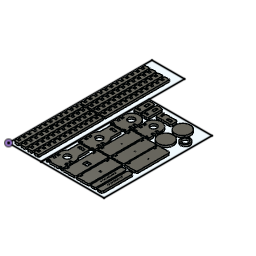
FinalFrameCAD (Autodesk Fusion 360 design; units mm, degrees)
Autodesk Fusion 360 part; units mm, degrees
note: some values were not read from the file. Chosen so that the rebuilt part matches the saved one: which bodies a step acts on.
sketch "Sketch1" plane through (0, 0, 0) normal (0, 0, 1) x (1, 0, 0)
  arc A0 (76.2, 342.8418) -> (-76.2, 342.8418) centre (0, 342.9) ccw
  line L0 (-45.085, 215.9582) -> (-45.085, 228.6582)
  line L1 (-45.085, 228.6582) -> (-63.5, 228.6582)
  line L2 (-63.5, 228.6582) -> (-63.5, 215.9582)
  line L3 (63.5, 215.9582) -> (63.5, 228.6582)
  line L4 (63.5, 228.6582) -> (45.085, 228.6582)
  line L5 (45.085, 228.6582) -> (45.085, 215.9582)
  line L6 (76.2, 215.9582) -> (63.5, 215.9582)
  line L7 (45.085, 215.9582) -> (-45.085, 215.9582)
  circle A1 centre (0, 342.9) radius 31.5595
  line L8 (76.2, 285.75) -> (50.8, 285.75)
  line L9 (50.8, 285.75) -> (50.8, 267.335)
  line L10 (50.8, 267.335) -> (76.2, 267.335)
  line L11 (76.2, 342.8418) -> (76.2, 323.85)
  line L12 (-76.2, 241.2418) -> (-76.2, 215.9582)
  line L13 (-76.2, 215.9582) -> (-63.5, 215.9582)
  line L14 (76.2, 305.435) -> (76.2, 285.75)
  line L15 (76.2, 267.335) -> (76.2, 215.9582)
  line L16 (76.2, 323.85) -> (50.8, 323.85)
  line L17 (50.8, 323.85) -> (50.8, 305.435)
  line L18 (50.8, 305.435) -> (76.2, 305.435)
  line L19 (-76.2, 323.85) -> (-50.8, 323.85)
  line L20 (-50.8, 323.85) -> (-50.8, 305.435)
  line L21 (-50.8, 305.435) -> (-76.2, 305.435)
  line L22 (-76.2, 285.75) -> (-50.8, 285.75)
  line L23 (-50.8, 285.75) -> (-50.8, 267.335)
  line L24 (-50.8, 267.335) -> (-76.2, 267.335)
  line L25 (-76.2, 323.85) -> (-76.2, 342.8418)
  line L26 (-76.2, 241.2418) -> (-76.2, 267.335)
  line L27 (-76.2, 285.75) -> (-76.2, 305.435)
  line L28 (279.4, 819.15) -> (254, 819.15)
  line L29 (266.7, 762.0582) -> (248.285, 762.0582)
  circle A2 centre (203.2, 876.3) radius 31.5595
  line L30 (254, 800.735) -> (279.4, 800.735)
  line L31 (279.4, 876.2418) -> (279.4, 857.25)
  line L32 (127, 749.3582) -> (139.7, 749.3582)
  line L33 (248.285, 762.0582) -> (248.285, 749.3582)
  line L34 (279.4, 857.25) -> (254, 857.25)
  line L35 (248.285, 749.3582) -> (158.115, 749.3582)
  line L36 (279.4, 838.835) -> (279.4, 819.15)
  line L37 (279.4, 800.735) -> (279.4, 749.3582)
  line L38 (254, 857.25) -> (254, 838.835)
  line L39 (254, 819.15) -> (254, 800.735)
  line L40 (152.4, 819.15) -> (152.4, 800.735)
  line L41 (127, 774.6418) -> (127, 749.3582)
  line L42 (152.4, 857.25) -> (152.4, 838.835)
  line L43 (139.7, 762.0582) -> (139.7, 749.3582)
  line L44 (158.115, 749.3582) -> (158.115, 762.0582)
  line L45 (127, 857.25) -> (127, 876.2418)
  line L46 (127, 819.15) -> (152.4, 819.15)
  line L47 (127, 819.15) -> (127, 838.835)
  line L48 (279.4, 749.3582) -> (266.7, 749.3582)
  line L49 (158.115, 762.0582) -> (139.7, 762.0582)
  line L50 (266.7, 749.3582) -> (266.7, 762.0582)
  line L51 (127, 857.25) -> (152.4, 857.25)
  line L52 (152.4, 838.835) -> (127, 838.835)
  line L53 (152.4, 800.735) -> (127, 800.735)
  line L54 (127, 774.6418) -> (127, 800.735)
  line L55 (254, 838.835) -> (279.4, 838.835)
  line L56 (203.2, 1003.1095) -> (228.6, 1003.1095)
  line L57 (228.6, 1003.1095) -> (228.6, 1021.5245)
  line L58 (228.6, 1021.5245) -> (203.2, 1021.5245)
  line L59 (177.8, 1021.5245) -> (203.2, 1021.5245)
  line L60 (203.2, 1003.1095) -> (177.8, 1003.1095)
  line L61 (177.8, 1003.1095) -> (177.8, 1021.5245)
  line L62 (152.4, 1021.5245) -> (152.4, 933.0961)
  line L63 (254, 1021.5245) -> (254, 933.0961)
  line L64 (152.4, 1021.5245) -> (152.4, 1046.9245)
  line L65 (152.4, 1046.9245) -> (254, 1046.9245)
  line L66 (254, 1046.9245) -> (254, 1021.5245)
  arc A3 (279.4, 876.2418) -> (254, 933.0961) centre (203.2, 876.3) ccw
  arc A4 (152.4, 933.0961) -> (127, 876.2418) centre (203.2, 876.3) ccw
  line L67 (590.55, 1066.8) -> (730.25, 1066.8)
  line L68 (812.8, 1066.8) -> (812.8, 1016)
  line L69 (812.8, 1016) -> (508, 1016)
  line L70 (508, 1016) -> (508, 1066.8)
  line L71 (508, 1066.8) -> (590.55, 1066.8)
  line L72 (730.25, 1066.8) -> (812.8, 1066.8)
  circle A5 centre (590.55, 1038.6277) radius 3.8735
  circle A6 centre (666.75, 1038.6277) radius 3.8735
  circle A7 centre (606.425, 1038.6277) radius 3.8735
  circle A8 centre (682.625, 1038.6277) radius 3.8735
  circle A9 centre (622.3, 1038.6277) radius 3.8735
  circle A10 centre (698.5, 1038.6277) radius 3.8735
  circle A11 centre (638.175, 1038.6277) radius 3.8735
  circle A12 centre (714.375, 1038.6277) radius 3.8735
  circle A13 centre (654.05, 1038.6277) radius 3.8735
  circle A14 centre (730.25, 1038.6277) radius 3.8735
  dimension "d55" = 152.4
  dimension "d58" = 101.6
  dimension "d59" = 18.415
  dimension "d60" = 12.7
  dimension "d61" = 12.7
  dimension "d62" = 18.415
  dimension "d63" = 12.7
  dimension "d64" = 12.7
  dimension "d195" = 63.119
  dimension "d197" = 25.4
  dimension "d198" = 18.415
  dimension "d199" = 25.4
  dimension "d200" = 18.415
  dimension "d264" = 152.4
  dimension "d265" = 101.6
  dimension "d266" = 18.415
  dimension "d267" = 12.7
  dimension "d268" = 12.7
  dimension "d269" = 18.415
  dimension "d270" = 12.7
  dimension "d271" = 12.7
  dimension "d272" = 63.119
  dimension "d273" = 25.4
  dimension "d274" = 18.415
  dimension "d275" = 25.4
  dimension "d276" = 18.415
  dimension "d279" = 25.4
  dimension "d280" = 18.415
  dimension "d281" = 25.4
  dimension "d282" = 25.4
  dimension "d283" = 304.8
  dimension "d284" = 50.8
  dimension "d286" = 7.747
  dimension "d287" = 7.747
  dimension "d288" = 7.747
  dimension "d289" = 7.747
  dimension "d290" = 7.747
  dimension "d291" = 7.747
  dimension "d292" = 7.747
  dimension "d293" = 7.747
  dimension "d294" = 7.747
  dimension "d295" = 7.747
  constraint perpendicular L6 L26
  constraint perpendicular L6 L14
  constraint coincident L2.end L6
  constraint perpendicular L1 L2
  constraint perpendicular L0 L6
  constraint perpendicular L0 L1
  constraint coincident L5.end L6
  constraint collinear L6 L7
  constraint perpendicular L5 L7
  constraint perpendicular L4 L5
  constraint concentric A0 A1
  constraint horizontal L8
  constraint vertical L9
  constraint horizontal L10
  constraint parallel L11 L14
  constraint parallel L12 L26
  constraint perpendicular L2 L13
  constraint collinear L14 L15
  constraint horizontal L16
  constraint vertical L17
  constraint horizontal L18
  constraint collinear L25 L26
  constraint perpendicular L48 L54
  constraint perpendicular L36 L48
  constraint coincident L32.end L48
  constraint perpendicular L43 L49
  constraint perpendicular L44 L48
  constraint perpendicular L44 L49
  constraint coincident L33.end L48
  constraint collinear L35 L48
  constraint perpendicular L33 L35
  constraint perpendicular L29 L33
  constraint concentric A2 A3
  constraint horizontal L28
  constraint vertical L39
  constraint horizontal L30
  constraint parallel L31 L36
  constraint parallel L41 L54
  constraint perpendicular L32 L43
  constraint collinear L36 L37
  constraint horizontal L34
  constraint vertical L38
  constraint horizontal L55
  constraint collinear L45 L54
  constraint horizontal L56
  constraint vertical L57
  constraint horizontal L58
  constraint coincident L62.end A3
  constraint concentric A3 A4
  constraint horizontal L67
  constraint vertical L68
  constraint horizontal L69
  constraint vertical L70
  constraint horizontal L71
  constraint horizontal L72
  constraint equal L71 L72
  measures "d55" diameter of A0
  measures "d58" distance of A0.end L12.start
  measures "d59" distance of L2.end L0.start
  measures "d60" distance of L2.end L1.end
  measures "d61" distance of L2 L26
  measures "d62" distance of L5.end L3.start
  measures "d63" distance of L5.end L4.end
  measures "d64" distance of L3 L14
  measures "d195" diameter of A1
  measures "d197" distance of L8.start L8.end
  measures "d198" distance of L8.start L10.end
  measures "d199" distance of L16.end L11.end
  measures "d200" distance of L14.start L11.end
  measures "d264" diameter of A3
  measures "d265" distance of L45.end L41.start
  measures "d266" distance of L35.end L32.end
  measures "d267" distance of L43.start L32.end
  measures "d268" distance of L43 L54
  measures "d269" distance of L48.end L33.end
  measures "d270" distance of L29.end L33.end
  measures "d271" distance of L36 L50
  measures "d272" diameter of A2
  measures "d273" distance of L28.end L28.start
  measures "d274" distance of L30.end L28.start
  measures "d275" distance of L31.end L34.end
  measures "d276" distance of L31.end L36.start
  measures "d279" distance of L56.start L56.end
  measures "d280" distance of L56.start L58.end
  measures "d281" distance of L57.end L63.start
  measures "d282" distance of L59.start L62.start
  measures "d283" distance of L70.end L68.start
  measures "d284" distance of L70.end L69.end
  measures "d286" diameter of A5
  measures "d287" diameter of A6
  measures "d288" diameter of A7
  measures "d289" diameter of A8
  measures "d290" diameter of A9
  measures "d291" diameter of A10
  measures "d292" diameter of A11
  measures "d293" diameter of A12
  measures "d294" diameter of A13
  measures "d295" diameter of A14
sketch "Sketch2" plane through (0, 0, 0) normal (0, 0, 1) x (1, 0, 0)
  line L0 (628.015, -50.8) -> (628.015, -101.6)
  line L1 (628.015, -101.6) -> (0, -101.6)
  line L2 (0, -101.6) -> (0, -50.8)
  line L3 (43.815, -50.8) -> (43.815, -76.2)
  line L4 (43.815, -76.2) -> (25.4, -76.2)
  line L5 (25.4, -76.2) -> (25.4, -50.8)
  line L6 (94.615, -50.8) -> (94.615, -76.2)
  line L7 (94.615, -76.2) -> (76.2, -76.2)
  line L8 (76.2, -76.2) -> (76.2, -50.8)
  line L9 (145.415, -50.8) -> (145.415, -76.2)
  line L10 (145.415, -76.2) -> (127, -76.2)
  line L11 (127, -76.2) -> (127, -50.8)
  line L12 (196.215, -50.8) -> (196.215, -76.2)
  line L13 (196.215, -76.2) -> (177.8, -76.2)
  line L14 (177.8, -76.2) -> (177.8, -50.8)
  line L15 (247.015, -50.8) -> (247.015, -76.2)
  line L16 (247.015, -76.2) -> (228.6, -76.2)
  line L17 (228.6, -76.2) -> (228.6, -50.8)
  line L18 (297.815, -50.8) -> (297.815, -76.2)
  line L19 (297.815, -76.2) -> (279.4, -76.2)
  line L20 (279.4, -76.2) -> (279.4, -50.8)
  line L21 (348.615, -50.8) -> (348.615, -76.2)
  line L22 (348.615, -76.2) -> (330.2, -76.2)
  line L23 (330.2, -76.2) -> (330.2, -50.8)
  line L24 (399.415, -50.8) -> (399.415, -76.2)
  line L25 (399.415, -76.2) -> (381, -76.2)
  line L26 (381, -76.2) -> (381, -50.8)
  line L27 (450.215, -50.8) -> (450.215, -76.2)
  line L28 (450.215, -76.2) -> (431.8, -76.2)
  line L29 (431.8, -76.2) -> (431.8, -50.8)
  line L30 (43.815, -50.8) -> (43.815, -76.2)
  line L31 (43.815, -76.2) -> (25.4, -76.2)
  line L32 (25.4, -76.2) -> (25.4, -50.8)
  line L33 (501.015, -50.8) -> (501.015, -76.2)
  line L34 (501.015, -76.2) -> (482.6, -76.2)
  line L35 (482.6, -76.2) -> (482.6, -50.8)
  line L36 (551.815, -50.8) -> (551.815, -76.2)
  line L37 (551.815, -76.2) -> (533.4, -76.2)
  line L38 (533.4, -76.2) -> (533.4, -50.8)
  line L39 (602.615, -50.8) -> (602.615, -76.2)
  line L40 (602.615, -76.2) -> (584.2, -76.2)
  line L41 (584.2, -76.2) -> (584.2, -50.8)
  line L42 (0, -50.8) -> (25.4, -50.8)
  line L43 (43.815, -50.8) -> (76.2, -50.8)
  line L44 (94.615, -50.8) -> (127, -50.8)
  line L45 (145.415, -50.8) -> (177.8, -50.8)
  line L46 (196.215, -50.8) -> (228.6, -50.8)
  line L47 (247.015, -50.8) -> (279.4, -50.8)
  line L48 (297.815, -50.8) -> (330.2, -50.8)
  line L49 (348.615, -50.8) -> (381, -50.8)
  line L50 (399.415, -50.8) -> (431.8, -50.8)
  line L51 (450.215, -50.8) -> (482.6, -50.8)
  line L52 (501.015, -50.8) -> (533.4, -50.8)
  line L53 (551.815, -50.8) -> (584.2, -50.8)
  line L54 (602.615, -50.8) -> (628.015, -50.8)
  dimension "d166" = 628.015
  dimension "d167" = 50.8
  dimension "d168" = 18.415
  dimension "d169" = 25.4
  dimension "d170" = 25.4
  dimension "d171" = 18.415
  dimension "d172" = 25.4
  dimension "d173" = 18.415
  dimension "d174" = 25.4
  dimension "d175" = 18.415
  dimension "d176" = 25.4
  dimension "d177" = 18.415
  dimension "d178" = 25.4
  dimension "d179" = 18.415
  dimension "d180" = 25.4
  dimension "d181" = 18.415
  dimension "d182" = 25.4
  dimension "d183" = 18.415
  dimension "d184" = 25.4
  dimension "d185" = 18.415
  dimension "d186" = 25.4
  dimension "d187" = 18.415
  dimension "d188" = 25.4
  dimension "d189" = 18.415
  dimension "d190" = 25.4
  dimension "d191" = 18.415
  dimension "d192" = 25.4
  dimension "d193" = 18.415
  dimension "d194" = 25.4
  constraint horizontal L42
  constraint vertical L0
  constraint horizontal L1
  constraint vertical L2
  constraint vertical L3
  constraint horizontal L4
  constraint vertical L5
  constraint vertical L6
  constraint horizontal L7
  constraint vertical L8
  constraint vertical L9
  constraint horizontal L10
  constraint vertical L11
  constraint vertical L12
  constraint horizontal L13
  constraint vertical L14
  constraint vertical L15
  constraint horizontal L16
  constraint vertical L17
  constraint vertical L18
  constraint horizontal L19
  constraint vertical L20
  constraint vertical L21
  constraint horizontal L22
  constraint vertical L23
  constraint vertical L24
  constraint horizontal L25
  constraint vertical L26
  constraint vertical L27
  constraint horizontal L28
  constraint vertical L29
  constraint vertical L30
  constraint horizontal L31
  constraint vertical L32
  constraint vertical L33
  constraint horizontal L34
  constraint vertical L35
  constraint vertical L36
  constraint horizontal L37
  constraint vertical L38
  constraint vertical L39
  constraint horizontal L40
  constraint vertical L41
  constraint collinear L42 L43
  constraint collinear L43 L44
  constraint collinear L44 L45
  constraint collinear L45 L46
  constraint collinear L46 L47
  constraint collinear L47 L48
  constraint collinear L48 L49
  constraint collinear L49 L50
  constraint collinear L50 L51
  constraint collinear L51 L52
  constraint collinear L52 L53
  constraint collinear L53 L54
  measures "d166" distance of L2.end L0.start
  measures "d167" distance of L2.end L1.end
  measures "d168" distance of L5.end L3.start
  measures "d169" distance of L5.end L4.end
  measures "d170" distance of L2 L5
  measures "d171" distance of L6.start L8.end
  measures "d172" distance of L7.end L8.end
  measures "d173" distance of L9.start L11.end
  measures "d174" distance of L10.end L11.end
  measures "d175" distance of L12.start L14.end
  measures "d176" distance of L13.end L14.end
  measures "d177" distance of L15.start L17.end
  measures "d178" distance of L16.end L17.end
  measures "d179" distance of L18.start L20.end
  measures "d180" distance of L19.end L20.end
  measures "d181" distance of L21.start L23.end
  measures "d182" distance of L22.end L23.end
  measures "d183" distance of L24.start L26.end
  measures "d184" distance of L25.end L26.end
  measures "d185" distance of L27.start L29.end
  measures "d186" distance of L28.end L29.end
  measures "d187" distance of L3.start L5.end
  measures "d188" distance of L4.end L5.end
  measures "d189" distance of L33.start L35.end
  measures "d190" distance of L34.end L35.end
  measures "d191" distance of L36.start L38.end
  measures "d192" distance of L37.end L38.end
  measures "d193" distance of L39.start L41.end
  measures "d194" distance of L40.end L41.end
sketch "Sketch3" plane through (0, 0, 0) normal (0, 0, 1) x (1, 0, 0)
  line L0 (0, 0) -> (323.215, 0)
  line L1 (323.215, 0) -> (323.215, 117.3988)
  line L2 (0, 117.3988) -> (0, 0)
  line L3 (43.815, 117.3988) -> (43.815, 104.6988)
  line L4 (43.815, 104.6988) -> (25.4, 104.6988)
  line L5 (25.4, 104.6988) -> (25.4, 117.3988)
  line L6 (279.4, 104.6988) -> (279.4, 117.3988)
  line L7 (297.815, 117.3988) -> (297.815, 104.6988)
  line L8 (297.815, 104.6988) -> (279.4, 104.6988)
  line L9 (25.4, 117.3988) -> (0, 117.3988)
  line L10 (323.215, 117.3988) -> (297.815, 117.3988)
  line L11 (279.4, 117.3988) -> (43.815, 117.3988)
  circle A0 centre (161.6075, 51.1556) radius 7.747
  line L12 (660.4, 117.3988) -> (424.815, 117.3988)
  line L13 (704.215, 117.3988) -> (678.815, 117.3988)
  line L14 (424.815, 104.6988) -> (406.4, 104.6988)
  line L15 (406.4, 104.6988) -> (406.4, 117.3988)
  line L16 (424.815, 117.3988) -> (424.815, 104.6988)
  line L17 (406.4, 117.3988) -> (381, 117.3988)
  line L18 (381, 117.3988) -> (381, 0)
  line L19 (678.815, 104.6988) -> (660.4, 104.6988)
  line L20 (678.815, 117.3988) -> (678.815, 104.6988)
  line L21 (660.4, 104.6988) -> (660.4, 117.3988)
  line L22 (704.215, 0) -> (704.215, 117.3988)
  line L23 (381, 0) -> (704.215, 0)
  circle A1 centre (542.6075, 51.1556) radius 3.8735
  line L24 (1041.4, 117.3988) -> (805.815, 117.3988)
  line L25 (762, 0) -> (1085.215, 0)
  line L26 (1085.215, 0) -> (1085.215, 117.3988)
  line L27 (1041.4, 104.6988) -> (1041.4, 117.3988)
  line L28 (1059.815, 117.3988) -> (1059.815, 104.6988)
  line L29 (805.815, 117.3988) -> (805.815, 104.6988)
  line L30 (762, 117.3988) -> (762, 0)
  line L31 (805.815, 104.6988) -> (787.4, 104.6988)
  line L32 (787.4, 117.3988) -> (762, 117.3988)
  line L33 (787.4, 104.6988) -> (787.4, 117.3988)
  line L34 (1059.815, 104.6988) -> (1041.4, 104.6988)
  line L35 (1085.215, 117.3988) -> (1059.815, 117.3988)
  line L36 (944.5625, 30.2006) -> (902.6525, 30.2006)
  line L37 (902.6525, 30.2006) -> (902.6525, 72.1106)
  line L38 (902.6525, 72.1106) -> (944.5625, 72.1106)
  line L39 (944.5625, 72.1106) -> (944.5625, 30.2006)
  line L40 (944.5625, 30.2006) -> (902.6525, 72.1106) construction
  line L41 (902.6525, 30.2006) -> (944.5625, 72.1106) construction
  point P0 (381, 0)
  point P1 (381, 0)
  point P2 (762, 0)
  point P3 (762, 0)
  point P4 (923.6075, 51.1556)
  dimension "d201" = 323.215
  dimension "d202" = 117.3988
  dimension "d203" = 18.415
  dimension "d204" = 12.7
  dimension "d205" = 25.4
  dimension "d206" = 18.415
  dimension "d207" = 12.7
  dimension "d209" = 15.494
  dimension "d211" = 323.215
  dimension "d212" = 117.3988
  dimension "d213" = 18.415
  dimension "d214" = 12.7
  dimension "d215" = 25.4
  dimension "d216" = 18.415
  dimension "d217" = 12.7
  dimension "d221" = 7.747
  dimension "d222" = 323.215
  dimension "d223" = 117.3988
  dimension "d224" = 18.415
  dimension "d225" = 12.7
  dimension "d226" = 25.4
  dimension "d227" = 18.415
  dimension "d228" = 12.7
  dimension "d232" = 41.91
  dimension "d233" = 41.91
  constraint horizontal L0
  constraint vertical L1
  constraint horizontal L10
  constraint vertical L2
  constraint coincident L0.start L2.end
  constraint vertical L3
  constraint horizontal L4
  constraint vertical L5
  constraint coincident L5.end L10
  constraint vertical L7
  constraint horizontal L8
  constraint vertical L6
  constraint collinear L9 L10
  constraint collinear L10 L11
  constraint horizontal L23
  constraint vertical L22
  constraint horizontal L13
  constraint vertical L18
  constraint coincident P1 P0
  constraint vertical L16
  constraint horizontal L14
  constraint vertical L15
  constraint coincident L15.end L13
  constraint vertical L20
  constraint horizontal L19
  constraint vertical L21
  constraint collinear L13 L17
  constraint collinear L12 L13
  constraint horizontal L25
  constraint vertical L26
  constraint horizontal L35
  constraint vertical L30
  constraint coincident P3 P2
  constraint vertical L29
  constraint horizontal L31
  constraint vertical L33
  constraint coincident L32.start L35
  constraint vertical L28
  constraint horizontal L34
  constraint vertical L27
  constraint collinear L32 L35
  constraint collinear L24 L35
  constraint horizontal L36
  constraint perpendicular L36 L37
  constraint parallel L36 L38
  constraint parallel L37 L39
  constraint coincident L40 P4
  constraint coincident L41 P4
  measures "d201" distance of L0.start L0.end
  measures "d202" distance of L0.start L2.start
  measures "d203" distance of L5.end L3.start
  measures "d204" distance of L5.end L4.end
  measures "d205" distance of L2 L5
  measures "d206" distance of L7.start L6.end
  measures "d207" distance of L6.end L6.start
  measures "d209" diameter of A0
  measures "d211" distance of L22.start P1
  measures "d212" distance of L17.end P1
  measures "d213" distance of L12.end L15.end
  measures "d214" distance of L15.end L14.end
  measures "d215" distance of L15 L18
  measures "d216" distance of L12.start L13.end
  measures "d217" distance of L12.start L19.end
  measures "d221" diameter of A1
  measures "d222" distance of L25.end P3
  measures "d223" distance of L30.start P3
  measures "d224" distance of L24.end L32.start
  measures "d225" distance of L32.start L31.end
  measures "d226" distance of L30 L33
  measures "d227" distance of L24.start L28.start
  measures "d228" distance of L24.start L27.start
  measures "d232" distance of L37.end L38.end
  measures "d233" distance of L36.end L37.end
sketch "Sketch4" plane through (0, 0, 0) normal (0, 0, 1) x (1, 0, 0)
  circle A0 centre (161.6075, 51.1556) radius 72.771
  line L0 (161.6075, 123.9266) -> (161.6075, 117.3988)
  point P0 (161.6075, 51.1556)
  point P1 (161.6075, 123.9266)
  point P2 (161.6075, 117.3988)
  dimension "d234" = 145.542
  constraint coincident P0 A0.centre
  constraint coincident P1 L0.start
  constraint coincident P2 L0.end
  measures "d234" diameter of A0
extrude "Extrude2" add sketch "Sketch1" sketch "Sketch2" sketch "Sketch3" along normal blind 18.415 of sketch 2 of sketch 3 makes body 1 at (66.0066, 51.1903, 0) makes body 2 at (319.405, -93.1333, 0) makes body 3 at (0.7861, 282.0329, 0) makes body 4 at (637.0124, 51.7273, 0) makes body 5 at (1023.7258, 44.9665, 0) makes body 6 at (202.4139, 971.3301, 0) makes body 7 at (534.2255, 1040.4759, 0)
copy_body "CopyPasteBodies24" bodies 2 makes body 8
move_body "Move36" bodies 8 to x (1, 0, 0) y (0, 1, 0) z (0, 0, 1) at (685.8, 0, 0)
move_body "Move37" bodies 3 to x (1, 0, 0) y (0, 1, 0) z (0, 0, 1) at (838.2, 0, 0)
move_body "Move38" bodies 5 to x (1, 0, 0) y (0, 1, 0) z (0, 0, 1) at (-762, 165.1, 0)
copy_body "CopyPasteBodies25" bodies 4 makes body 9
move_body "Move39" bodies 9 to x (1, 0, 0) y (0, 1, 0) z (0, 0, 1) at (0, 165.1, 0)
move_body "Move40" bodies 3 to x (1, 0, 0) y (0, 1, 0) z (0, 0, 1) at (0, -215.9, 0)
copy_body "CopyPasteBodies26" bodies 3 makes body 10
move_body "Move41" bodies 10 to x (1, 0, 0) y (0, 1, 0) z (0, 0, 1) at (203.2, 0, 0)
move_body "Move42" bodies 8 to x (1, 0, 0) y (0, 1, 0) z (0, 0, 1) at (-685.8, 431.8, 0)
move_body "Move43" bodies 3 to x (1, 0, 0) y (0, 1, 0) z (0, 0, 1) at (0, -101.6, 0)
move_body "Move44" bodies 10 to x (1, 0, 0) y (0, 1, 0) z (0, 0, 1) at (0, 177.8, 0)
move_body "Move45" bodies 10 to x (-1, 0, 0) y (0, -1, 0) z (0, 0, 1) at (1879.6, 558.9164, 0)
move_body "Move46" bodies 3 to x (1, 0, 0) y (0, 1, 0) z (0, 0, 1) at (304.8, 228.6, 0)
move_body "Move47" bodies 2 to x (1, 0, 0) y (0, 1, 0) z (0, 0, 1) at (127, 12.7, 0)
copy_body "CopyPasteBodies27" bodies 2 makes body 11
move_body "Move48" bodies 11 to x (1, 0, 0) y (0, 1, 0) z (0, 0, 1) at (812.8, 0, 0)
move_body "Move49" bodies 8 to x (1, 0, 0) y (0, 1, 0) z (0, 0, 1) at (127, -546.1, 0)
copy_body "CopyPasteBodies28" bodies 8 makes body 12
move_body "Move50" bodies 12 to x (1, 0, 0) y (0, 1, 0) z (0, 0, 1) at (711.2, 0, 0)
move_body "Move51" bodies 11 to x (1, 0, 0) y (0, 1, 0) z (0, 0, 1) at (-101.6, 0, 0)
move_body "Move52" bodies 5 9 4 1 to x (1, 0, 0) y (0, 1, 0) z (0, 0, 1) at (50.8, 50.8, 0)
move_body "Move53" bodies 7 to x (1, 0, 0) y (0, 1, 0) z (0, 0, 1) at (1016, -1231.9, 0)
move_body "Move54" bodies 2 to x (1, 0, 0) y (0, 1, 0) z (0, 0, 1) at (50.8, 0, 0)
move_body "Move55" bodies 8 to x (1, 0, 0) y (0, 1, 0) z (0, 0, 1) at (50.8, 0, 0)
move_body "Move56" bodies 7 to x (1, 0, 0) y (0, 1, 0) z (0, 0, 1) at (-25.4, 0, 0)
move_body "Move57" bodies 10 to x (1, 0, 0) y (0, 1, 0) z (0, 0, 1) at (25.4, -127, 0)
move_body "Move58" bodies 3 to x (1, 0, 0) y (0, 1, 0) z (0, 0, 1) at (-279.4, 152.4, 0)
move_body "Move59" bodies 6 to x (0, -1, 0) y (1, 0, 0) z (0, 0, 1) at (-698.5, 647.7, 0)
copy_body "CopyPasteBodies29" bodies 6 makes body 13
move_body "Move60" bodies 13 to x (1, 0, 0) y (0, 1, 0) z (0, 0, 1) at (381, 0, 0)
fillet "Fillet3" radius 12.7 24 edges at (374.015, 50.8, 9.2075) (50.8, 50.8, 9.2075) (177.8, -38.1, 9.2075) (805.815, -38.1, 9.2075) (755.015, 50.8, 9.2075) (431.8, 50.8, 9.2075) (50.8, 215.9, 9.2075) (374.015, 215.9, 9.2075) (177.8, -165.1, 9.2075) (805.815, -165.1, 9.2075) (431.8, 215.9, 9.2075) (755.015, 215.9, 9.2075) (348.4245, 393.7, 9.2075) (348.4245, 495.3, 9.2075) (1498.6, -165.1, 9.2075) (1498.6, -215.9, 9.2075) (1803.4, -215.9, 9.2075) (1803.4, -165.1, 9.2075) (838.2, -38.1, 9.2075) (1466.215, -38.1, 9.2075) (838.2, -165.1, 9.2075) (1466.215, -165.1, 9.2075) (729.4245, 393.7, 9.2075) (729.4245, 495.3, 9.2075) on bodies 1 2 4 5 6 7 8 9 11 12 13
sketch "Sketch6" plane through (0, 0, 0) normal (0, 0, 1) x (1, 0, 0)
  line L0 (0, 0) -> (315.9125, 0)
  line L1 (315.9125, 0) -> (315.9125, 1390.65)
  line L2 (315.9125, 1390.65) -> (0, 1390.65)
  line L3 (0, 1390.65) -> (0, 0)
  line L4 (315.9125, 0) -> (925.5125, 0)
  line L5 (925.5125, 0) -> (925.5125, 1047.75)
  line L6 (925.5125, 1047.75) -> (315.9125, 1047.75)
  line L7 (315.9125, 1047.75) -> (315.9125, 0)
  dimension "d305" = 315.9125
  dimension "d306" = 1390.65
  dimension "d307" = 609.6
  dimension "d308" = 1047.75
  constraint horizontal L0
  constraint vertical L1
  constraint horizontal L2
  constraint vertical L3
  constraint coincident L0.start L3.end
  constraint horizontal L4
  constraint vertical L5
  constraint horizontal L6
  constraint vertical L7
  measures "d305" distance of L0.start L0.end
  measures "d306" distance of L0.start L2.end
  measures "d307" distance of L0.end L4.end
  measures "d308" distance of L0.end L6.end
move_body "Move66" bodies 6 5 1 4 9 13 3 10 to x (1, 0, 0) y (0, 1, 0) z (0, 0, 1) at (939.8, 0, 0)
move_body "Move67" bodies 2 8 11 12 to x (0, 1, 0) y (-1, 0, 0) z (0, 0, 1) at (-19.685, -132.715, 0)
move_body "Move68" bodies 2 8 to x (1, 0, 0) y (0, 1, 0) z (0, 0, 1) at (0, -19.05, 0)
move_body "Move69" bodies 8 to x (1, 0, 0) y (0, 1, 0) z (0, 0, 1) at (-63.5, 0, 0)
move_body "Move70" bodies 12 to x (1, 0, 0) y (0, 1, 0) z (0, 0, 1) at (0, -685.8, 0)
move_body "Move71" bodies 2 8 12 to x (1, 0, 0) y (0, 1, 0) z (0, 0, 1) at (0, 5.715, 0)
move_body "Move72" bodies 2 8 12 to x (1, 0, 0) y (0, 1, 0) z (0, 0, 1) at (5.715, -6.35, 0)
move_body "Move73" bodies 2 8 12 to x (1, 0, 0) y (0, 1, 0) z (0, 0, 1) at (1.27, 0, 0)
move_body "Move74" bodies 11 to x (1, 0, 0) y (0, 1, 0) z (0, 0, 1) at (203.2, -685.8, 0)
move_body "Move75" bodies 11 to x (1, 0, 0) y (0, 1, 0) z (0, 0, 1) at (-5.715, 0, 0)
move_body "Move76" bodies 11 to x (1, 0, 0) y (0, 1, 0) z (0, 0, 1) at (0, 5.715, 0)
move_body "Move77" bodies 12 to x (1, 0, 0) y (0, 1, 0) z (0, 0, 1) at (0, 6.35, 0)
move_body "Move78" bodies 6 5 1 4 9 13 to x (0, 1, 0) y (-1, 0, 0) z (0, 0, 1) at (882.2961, -958.4961, 0)
move_body "Move79" bodies 13 6 5 9 4 1 to x (1, 0, 0) y (0, 1, 0) z (0, 0, 1) at (-20.2946, 0, 0)
move_body "Move80" bodies 13 9 4 1 5 6 to x (1, 0, 0) y (0, 1, 0) z (0, 0, 1) at (0, -8.4582, 0)
move_body "Move81" bodies 6 5 1 to x (1, 0, 0) y (0, 1, 0) z (0, 0, 1) at (0, 1.7018, 0)
move_body "Move82" bodies 13 9 4 to x (1, 0, 0) y (0, 1, 0) z (0, 0, 1) at (0, -34.798, 0)
move_body "Move83" bodies 9 4 to x (1, 0, 0) y (0, 1, 0) z (0, 0, 1) at (0, 4.1148, 0)
move_body "Move84" bodies 13 to x (1, 0, 0) y (0, 1, 0) z (0, 0, 1) at (0, -21.5392, 0)
move_body "Move85" bodies 13 9 4 to x (1, 0, 0) y (0, 1, 0) z (0, 0, 1) at (0, -12.7, 0)
move_body "Move86" bodies 9 5 to x (1, 0, 0) y (0, 1, 0) z (0, 0, 1) at (-9.4488, 0, 0)
move_body "Move87" bodies 9 5 to x (1, 0, 0) y (0, 1, 0) z (0, 0, 1) at (-12.7152, 0, 0)
move_body "Move88" bodies 1 4 to x (1, 0, 0) y (0, 1, 0) z (0, 0, 1) at (-44.4754, 0, 0)
move_body "Move89" bodies 4 1 to x (1, 0, 0) y (0, 1, 0) z (0, 0, 1) at (-12.7, 0, 0)
move_body "Move90" bodies 10 3 to x (1, 0, 0) y (0, 1, 0) z (0, 0, 1) at (-1701.8, 635, 0)
move_body "Move91" bodies 3 10 to x (1, 0, 0) y (0, 1, 0) z (0, 0, 1) at (0, -19.05, 0)
move_body "Move92" bodies 3 to x (1, 0, 0) y (0, 1, 0) z (0, 0, 1) at (0, -12.7, 0)
move_body "Move93" bodies 7 to x (0, -1, 0) y (1, 0, 0) z (0, 0, 1) at (431.8, 2514.6, 0)
move_body "Move94" bodies 3 to x (1, 0, 0) y (0, 1, 0) z (0, 0, 1) at (330.2, -228.6, 0)
move_body "Move95" bodies 3 to x (1, 0, 0) y (0, 1, 0) z (0, 0, 1) at (-14.3002, 0, 0)
move_body "Move96" bodies 3 to x (1, 0, 0) y (0, 1, 0) z (0, 0, 1) at (0, -8.1788, 0)
move_body "Move97" bodies 10 to x (-1, 0, 0) y (0, -1, 0) z (0, 0, 1) at (681.7897, 1577.918, 0)
move_body "Move98" bodies 10 to x (1, 0, 0) y (0, 1, 0) z (0, 0, 1) at (0, -10.7442, 0)
move_body "Move99" bodies 10 to x (1, 0, 0) y (0, 1, 0) z (0, 0, 1) at (2.413, 0, 0)
move_body "Move100" bodies 7 to x (1, 0, 0) y (0, 1, 0) z (0, 0, 1) at (558.8, -685.8, 0)
move_body "Move101" bodies 7 to x (1, 0, 0) y (0, 1, 0) z (0, 0, 1) at (-7.9756, 0, 0)
copy_body "CopyPasteBodies33" bodies 2 8 12 11 makes body 14 makes body 15 makes body 16 makes body 17
move_body "Move102" bodies 14 15 16 17 to x (1, 0, 0) y (0, 1, 0) z (0, 0, 1) at (0, 660.4, 0)
move_body "Move103" bodies 14 15 16 17 to x (1, 0, 0) y (0, 1, 0) z (0, 0, 1) at (0, -19.685, 0)
copy_body "CopyPasteBodies34" bodies 7 makes body 18
move_body "Move104" bodies 18 to x (1, 0, 0) y (0, 1, 0) z (0, 0, 1) at (63.5, 0, 0)
sketch "Sketch7" plane through (0, 0, 0) normal (0, 0, 1) x (1, 0, 0)
  line L0 (835.025, 635) -> (854.075, 635)
  line L1 (854.075, 635) -> (854.075, 593.725)
  line L2 (854.075, 593.725) -> (835.025, 593.725)
  line L3 (835.025, 593.725) -> (835.025, 635)
  line L4 (812.8, 660.4) -> (876.3, 660.4)
  line L5 (876.3, 660.4) -> (876.3, 508)
  line L6 (876.3, 508) -> (812.8, 508)
  line L7 (812.8, 533.4) -> (850.9, 533.4)
  line L8 (850.9, 533.4) -> (850.9, 546.1)
  line L9 (850.9, 546.1) -> (812.8, 546.1)
  line L10 (812.8, 508) -> (812.8, 533.4)
  line L11 (812.8, 546.1) -> (812.8, 660.4)
  dimension "d309" = 19.05
  dimension "d310" = 41.275
  dimension "d311" = 22.225
  dimension "d312" = 25.4
  dimension "d313" = 38.1
  constraint horizontal L0
  constraint vertical L1
  constraint horizontal L2
  constraint vertical L3
  constraint horizontal L4
  constraint vertical L5
  constraint horizontal L6
  constraint vertical L10
  constraint horizontal L7
  constraint vertical L8
  constraint horizontal L9
  constraint collinear L10 L11
  measures "d309" distance of L0.start L0.end
  measures "d310" distance of L0.start L2.end
  measures "d311" distance of L3 L10
  measures "d312" distance of L0 L4
  measures "d313" distance of L7.start L7.end
extrude "Extrude3" add sketch "Sketch7" along normal blind 18.415 separate body makes body 19
fillet "Fillet4" radius 12.7 4 edges at (812.8, 508, 9.2075) (876.3, 508, 9.2075) (876.3, 660.4, 9.2075) (812.8, 660.4, 9.2075) on bodies 19
copy_body "CopyPasteBodies35" bodies 19 makes body 20
move_body "Move105" bodies 20 to x (1, 0, 0) y (0, 1, 0) z (0, 0, 1) at (76.2, 0, 0)
move_body "Move106" bodies 19 20 to x (1, 0, 0) y (0, 1, 0) z (0, 0, 1) at (-469.9, 355.6, 0)
copy_body "CopyPasteBodies36" bodies 4 makes body 21
move_body "Move107" bodies 21 to x (1, 0, 0) y (0, 1, 0) z (0, 0, 1) at (127, 0, 0)
copy_body "CopyPasteBodies37" bodies 21 makes body 22
sketch "Sketch8" plane through (0, 0, 0) normal (0, 0, 1) x (1, 0, 0)
  circle A0 centre (762, 889) radius 72.771
  circle A1 centre (990.6, 889) radius 31.623
  circle A2 centre (990.6, 889) radius 44.45
  dimension "d318" = 145.542
  dimension "d324" = 63.246
  dimension "d325" = 88.9
  constraint concentric A1 A2
  measures "d318" diameter of A0
  measures "d324" diameter of A1
  measures "d325" diameter of A2
extrude "Extrude5" add sketch "Sketch8" along normal blind 18.415 separate body makes body 23 at (726.6922, 908.1406, 0) makes body 24 at (1034.9947, 886.7843, 12.2767)
move_body "Move110" bodies 23 to x (1, 0, 0) y (0, 1, 0) z (0, 0, 1) at (0, -101.6, 0)
move_body "Move111" bodies 23 to x (1, 0, 0) y (0, 1, 0) z (0, 0, 1) at (-12.7, -12.7, 0)
copy_body "CopyPasteBodies38" bodies 23 makes body 25
move_body "Move112" bodies 25 to x (1, 0, 0) y (0, 1, 0) z (0, 0, 1) at (-38.1, 165.1, 0)
copy_body "CopyPasteBodies39" bodies 20 makes body 26
move_body "Move113" bodies 26 to x (1, 0, 0) y (0, 1, 0) z (0, 0, 1) at (381, -12.7, 0)
move_body "Move114" bodies 26 to x (0, -1, 0) y (1, 0, 0) z (0, 0, 1) at (-349.25, 1784.35, 0)
move_body "Move115" bodies 25 to x (1, 0, 0) y (0, 1, 0) z (0, 0, 1) at (38.1, 0, 0)
move_body "Move116" bodies 24 to x (1, 0, 0) y (0, 1, 0) z (0, 0, 1) at (-133.35, -31.75, 0)
equation "notch = 0.6 in" comment "notch"
